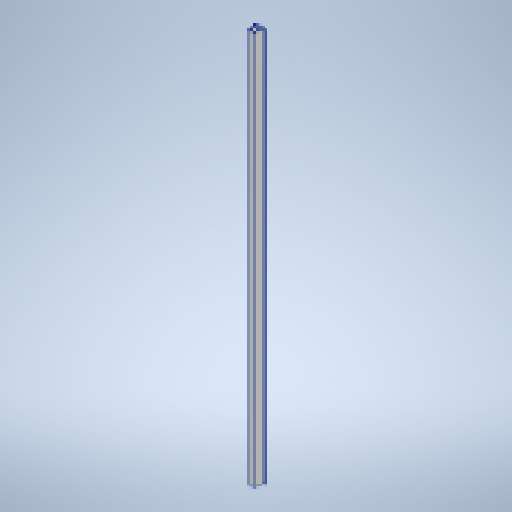
# Autodesk Inventor part: TrägerUI
Saved by Autodesk Inventor 2025 (Build 290162010, 162A)
## iProperties
Created: 2025-02-04
Part Number: TrägerUI
Material: Aluminium 6061, Katze
Document SubType Name: Modeling
Designer: Admin
Density: 2.7 g/cm^3
Appearance: Aluminium - flach(1)
Mass: 437.4 g
Surface Area: 1623.24 cm^2
Volume: 162 cm^3
Author: Admin
Autodesk Inventor part; units mm, degrees
ref_plane "YZ Plane" through (0, 0, 0) normal (1, 0, 0) x (0, 1, 0)
ref_plane "XZ Plane" through (0, 0, 0) normal (0, 1, 0) x (-1, 0, 0)
ref_plane "XY Plane" through (0, 0, 0) normal (0, 0, 1) x (1, 0, 0)
sketch "Skizze1" plane through (0, 0, 0) normal (0, 0, 1) x (1, 0, 0)
  line L0 (0, 0) -> (30, 0)
  line L1 (30, 0) -> (30, -2)
  line L2 (30, -2) -> (0, -2)
  line L3 (0, -2) -> (0, 0)
  line L4 (7.5, -2) -> (9.5, -2)
  line L5 (9.5, -2) -> (9.5, -22)
  line L6 (9.5, -22) -> (7.5, -22)
  line L7 (7.5, -22) -> (7.5, -2)
  line L8 (9.5, -22) -> (20.5, -22)
  line L9 (20.5, -22) -> (20.5, -20)
  line L10 (20.5, -20) -> (9.5, -20)
  line L11 (9.5, -20) -> (9.5, -22)
  line L12 (20.5, -22) -> (22.5, -22)
  line L13 (22.5, -22) -> (22.5, -2)
  line L14 (22.5, -2) -> (20.5, -2)
  line L15 (20.5, -2) -> (20.5, -22)
  line L16 (15, -20) -> (15, -2) construction
  point P0 (20.5, -2)
  point P1 (9.5, -2)
  dimension "d0" = 30
  dimension "d1" = 2
  dimension "d2" = 2
  dimension "d3" = 20
  dimension "d4" = 11
  dimension "d5" = 2
  dimension "d6" = 2
  dimension "d7" = 7.5
  dimension "d8" = 20.5
  dimension "d9" = 20
  dimension "d12" = 7.5
  constraints: 34 end point, 8 parallel, 4 horizontal, 4 perpendicular, 2 midpoint, 2 point on line, 1 vertical
  measures "d0" distance of L1.end L2.end
  measures "d1" distance of L0.end L1.end
  measures "d2" distance of L5.end L6.end
  measures "d3" distance of L4.end L5.end
  measures "d4" distance of L10.end L9.end
  measures "d5" distance of L9.end L8.end
  measures "d6" distance of L14.end L13.end
  measures "d7" distance from line of L2.end L7
  measures "d8" distance of L2.end L14.end
  measures "d9" vertical distance of L0.start L10.end
  measures "d12" distance from line of L13 L1.end
extrude "Extrusion1" add sketch "Skizze1" along normal blind 1000 contours L0 L1 L2 L3 | L2 L5 L6 L7 | L13 L12 L9 L15 L2 | L10 L9 L8 L5
